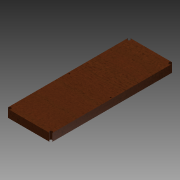
# Autodesk Inventor part: Mid
Saved by Autodesk Inventor 2015 (Build 190159000, 159)
## iProperties
Created: 2014-07-25
Part Number: Mid
Material: Wood (Walnut)
Document SubType Name: Modeling
Designer: Michael
Density: 0.55 g/cm^3
Appearance: Walnut - Natural Polished
Author: Michael
Autodesk Inventor part; units mm, degrees
ref_plane "YZ Plane" through (0, 0, 0) normal (1, 0, 0) x (0, 1, 0)
ref_plane "XZ Plane" through (0, 0, 0) normal (0, 1, 0) x (-1, 0, 0)
ref_plane "XY Plane" through (0, 0, 0) normal (0, 0, 1) x (1, 0, 0)
sketch "Sketch1" plane through (0, 0, 0) normal (0, 1, 0) x (-1, 0, 0)
  line L0 (-0.444, 225.316) -> (-86.169, 225.316)
  line L1 (-89.344, 222.141) -> (-89.344, -25.509)
  line L2 (-86.169, -28.684) -> (-0.444, -28.684)
  line L3 (2.731, -25.509) -> (2.731, 222.141)
  arc A0 (-86.169, -28.684) -> (-89.344, -25.509) centre (-86.169, -25.509) ccw
  arc A1 (-0.444, 225.316) -> (2.731, 222.141) centre (-0.444, 222.141) ccw
  arc A2 (-89.344, 222.141) -> (-86.169, 225.316) centre (-86.169, 222.141) ccw
  arc A3 (2.731, -25.509) -> (-0.444, -28.684) centre (-0.444, -25.509) ccw
  circle A4 centre (-0.444, 98.316) radius 1.4732
  circle A5 centre (-86.169, 98.316) radius 1.4732
  point P0 (0, 0)
  dimension "d2" = 6.35
  dimension "d3" = 6.35
  dimension "d4" = 6.35
  dimension "d5" = 6.35
  dimension "d7" = 2.9464
  dimension "d8" = 2.9464
  constraints: 8 end point, 8 point on circle, 6 centre point
  measures "d2" diameter of A0
  measures "d3" diameter of A1
  measures "d4" diameter of A2
  measures "d5" diameter of A3
  measures "d7" diameter of A4
  measures "d8" diameter of A5
extrude "Extrusion1" add sketch "Sketch1" along normal blind 15.875
body "Solid1"
